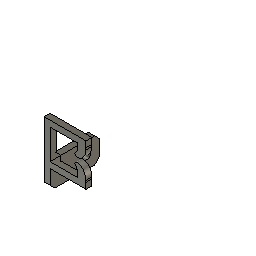
horizontal (Autodesk Fusion 360 design; units mm, degrees)
Autodesk Fusion 360 part; units mm, degrees
sketch "rail-body" plane through (1.3, 0, 0) normal (1, 0, 0) x (0, 1, 0)
  line L0 (50.85, 4.575) -> (60, 4.575)
  line L1 (60, 4.575) -> (60, 14.775)
  line L2 (60, 14.775) -> (0, 14.775)
  line L3 (0, 14.775) -> (0, -14.775)
  line L4 (0, -14.775) -> (60, -14.775)
  line L5 (60, -14.775) -> (60, -4.575)
  line L6 (60, -4.575) -> (50.85, -4.575)
  line L7 (50.85, -4.575) -> (50.85, 4.575)
  line L8 (30.85, 4.575) -> (40, 4.575)
  line L9 (40, 4.575) -> (40, -4.575)
  line L10 (40, -4.575) -> (30.85, -4.575)
  line L11 (30.85, -4.575) -> (30.85, 4.575)
  line L12 (10.85, 4.575) -> (20, 4.575)
  line L13 (20, 4.575) -> (20, -4.575)
  line L14 (20, -4.575) -> (10.85, -4.575)
  line L15 (10.85, -4.575) -> (10.85, 4.575)
  circle A0 centre (15.425, 0) radius 3.5
  line L16 (10.85, 4.575) -> (20, -4.575) construction
  line L17 (20, 4.575) -> (10.85, -4.575) construction
  line L18 (30.85, 4.575) -> (40, -4.575) construction
  line L19 (40, 4.575) -> (30.85, -4.575) construction
  circle A1 centre (35.425, 0) radius 3.5
  line L20 (4.85, 10.575) -> (46, 10.575)
  line L21 (46, 10.575) -> (46, -10.575)
  line L22 (46, -10.575) -> (4.85, -10.575)
  line L23 (4.85, -10.575) -> (4.85, 10.575)
  point P0 (15.425, 0)
  point P1 (35.425, 0)
  dimension "d28" = 7
  dimension "d30" = 7
  dimension "d31" = 6
  dimension "d32" = 6
  dimension "d33" = 6
  dimension "d34" = 6
  constraint coincident L12.start L15.end
  constraint coincident L13.end L14.start
  constraint coincident L12.end L13.start
  constraint coincident L14.end L15.start
  constraint midpoint L16 P0
  constraint coincident P0 A0.centre
  constraint coincident L8.start L11.end
  constraint coincident L9.end L10.start
  constraint coincident L8.end L9.start
  constraint coincident L10.end L11.start
  constraint midpoint L18 P1
  constraint coincident P1 A1.centre
  constraint horizontal L20
  constraint vertical L21
  constraint horizontal L22
  constraint vertical L23
  measures "d28" diameter of A0
  measures "d30" diameter of A1
  measures "d31" distance of L15 L23
  measures "d32" distance of L9 L21
  measures "d33" distance of L14 L22
  measures "d34" distance of L12 L20
extrude "Extrude1" add sketch "rail-body" along normal blind 5 contours L8 L9 L10 L11 | L12 L13 L14 L15 | L20 L21 L22 L23
sketch "cable-body" plane through (0, 4.85, 0) normal (0, -1, 0) x (1, 0, 0)
  line L0 (1.3, 10.575) -> (1.3, -10.575)
  line L1 (1.3, -10.575) -> (6.3, -10.575)
  line L2 (6.3, -10.575) -> (6.3, 10.575)
  line L3 (6.3, 10.575) -> (1.3, 10.575)
  line L4 (6.3, 3.5) -> (6.3, -3.5)
  line L5 (6.3, 5.5) -> (36.3, 5.5)
  line L6 (1.3, 40.5) -> (36.3, 40.5)
  line L7 (6.3, 35.5) -> (36.3, 35.5)
  line L8 (6.3, 10.5) -> (6.3, 35.5)
  line L9 (6.3, 10.5) -> (36.3, 10.5)
  line L10 (1.3, 5.5) -> (1.3, 40.5)
  line L11 (36.3, 5.5) -> (36.3, 10.5)
  line L12 (36.3, 35.5) -> (36.3, 40.5)
  line L13 (6.3, 5.5) -> (1.3, 5.5) construction
  dimension "d51" = 2
  dimension "d53" = 35
  dimension "d55" = 35
  dimension "d56" = 5
  dimension "d57" = 5
  dimension "d58" = 5
  dimension "d59" = 35
  constraint coincident L2 L5.start
  constraint perpendicular L2 L5
  constraint parallel L6 L7
  constraint parallel L5 L9
  constraint vertical L10
  constraint coincident L0 L10.start
  constraint perpendicular L9 L11
  constraint perpendicular L6 L12
  constraint perpendicular L0 L13
  constraint coincident L10.start L13.end
  measures "d51" distance of L4.start L5.start
  measures "d53" distance of L0 L5.end
  measures "d55" distance of L10.start L6.start
  measures "d56" distance of L8 L10
  measures "d57" distance of L6 L7
  measures "d58" distance of L5 L9
  measures "d59" distance of L10 L12
sketch "hook-profile" plane through (0, 0, 0) normal (0, 1, 0) x (1, 0, 0)
  line L0 (6.3, -35.5) -> (36.3, -35.5)
  line L1 (36.3, -35.5) -> (36.3, -40.5)
  line L2 (6.3, -10.5) -> (6.3, -35.5)
  line L3 (6.3, -23) -> (36.2838, -23) construction
  line L4 (29.5303, -34) -> (36.3, -34)
  spline S0 degree 5 poles (36.3, -34) (36.2969, -33.8937) (36.2885, -33.6812) (36.2691, -33.3623) (36.2293, -32.9375) (36.1547, -32.4091) (36.0533, -31.8865) (35.9239, -31.373) (35.7665, -30.8717) (35.5835, -30.3849) (35.3795, -29.9139) (35.1598, -29.4591) (34.9292, -29.0202) (34.6901, -28.597) (34.4418, -28.1889) (34.1783, -27.7958) (33.8908, -27.4178) (33.5695, -27.0553) (33.2063, -26.7097) (32.7967, -26.3826) (32.3428, -26.0767) (31.8525, -25.7957) (31.3377, -25.5438) (30.8125, -25.3262) (30.291, -25.1489) (29.7863, -25.0187) (29.3079, -24.9432) (28.8625, -24.9299) (28.455, -24.9841) (28.0897, -25.108) (27.7716, -25.2988) (27.5068, -25.5475) (27.3024, -25.8403) (27.1648, -26.1605) (27.0993, -26.4904) (27.1085, -26.813) (27.1914, -27.1155) (27.3423, -27.3932) (27.5486, -27.6536) (27.7911, -27.9174) (28.0485, -28.2097) (28.3012, -28.5519) (28.5353, -28.9539) (28.7465, -29.4066) (28.936, -29.8899) (29.1067, -30.3823) (29.2596, -30.8681) (29.3893, -31.3469) (29.4813, -31.841) (29.5355, -32.3554) (29.5566, -32.8899) (29.554, -33.3294) (29.5446, -33.6634) (29.5355, -33.8876) (29.5303, -34) knots 0 0 0 0 0 0 0.02 0.04 0.06 0.08 0.1 0.12 0.14 0.16 0.18 0.2 0.22 0.24 0.26 0.28 0.3 0.32 0.34 0.36 0.38 0.4 0.42 0.44 0.46 0.48 0.5 0.52 0.54 0.56 0.58 0.6 0.62 0.64 0.66 0.68 0.7 0.72 0.74 0.76 0.78 0.8 0.82 0.84 0.86 0.88 0.9 0.92 0.94 0.96 0.98 1 1 1 1 1 1
  line L5 (36.3614, -36.1245) -> (36.2386, -31.8755)
  line L6 (28.7615, -29.0469) -> (29.842, -33.0275)
  line L7 (29.6357, -31.738) -> (29.4248, -36.262)
  line L8 (29.5815, -35.5) -> (36.2971, -35.5)
  line L9 (36.3, -35.5) -> (36.3, -33.7789)
  line L10 (29.5303, -34) -> (29.5303, -35.5)
  point P0 (27.3103, -27.3155)
  point P1 (34.6614, -28.5561)
  point P2 (28.2897, -28.5561)
  point P3 (33.0561, -26.5973)
  point P4 (35.8142, -31.0372)
  point P5 (27.1797, -26.1729)
  point P6 (30.1832, -25.1282)
  point P7 (28.0938, -25.1282)
  point P8 (29.3018, -31.0372)
  dimension "d60" = 1.5
  constraint midpoint L2 L3.start
  constraint perpendicular L2 L3
  constraint coincident L4.start S0.end
  constraint horizontal L4
  constraint midpoint L4.end L5
  constraint midpoint P8 L6
  constraint midpoint L4.start L7
  constraint horizontal L8
  constraint collinear L0 L8
  constraint coincident L0.end L1.start
  constraint perpendicular L8 L9
  constraint coincident L4.end L9
  constraint coincident L0 L10.end
  constraint vertical L10
  measures "d60" distance of L4 L8
sketch "Sketch5" plane through (3.8, 4.85, 0) normal (0, -1, 0) x (1, 0, 0)
  line L0 (2.5, 35.5) -> (32.5, 35.5)
  line L1 (2.5, 10.5) -> (2.5, 35.5)
  line L2 (-2.5, 40.5) -> (32.5, 40.5)
  line L3 (32.5, 35.5) -> (32.5, 40.5)
  line L4 (-2.5, 5.5) -> (-2.5, 40.5)
  line L5 (2.5, 5.5) -> (-2.5, 5.5)
  line L6 (2.5, 5.5) -> (32.5, 5.5)
  line L7 (32.5, 5.5) -> (32.5, 10.5)
  line L8 (2.5, 10.5) -> (32.5, 10.5)
  spline S0 degree 5 poles (36.3, -34) (36.2969, -33.8937) (36.2885, -33.6812) (36.2691, -33.3623) (36.2293, -32.9375) (36.1547, -32.4091) (36.0533, -31.8865) (35.9239, -31.373) (35.7665, -30.8717) (35.5835, -30.3849) (35.3795, -29.9139) (35.1598, -29.4591) (34.9292, -29.0202) (34.6901, -28.597) (34.4418, -28.1889) (34.1783, -27.7958) (33.8908, -27.4178) (33.5695, -27.0553) (33.2063, -26.7097) (32.7967, -26.3826) (32.3428, -26.0767) (31.8525, -25.7957) (31.3377, -25.5438) (30.8125, -25.3262) (30.291, -25.1489) (29.7863, -25.0187) (29.3079, -24.9432) (28.8625, -24.9299) (28.455, -24.9841) (28.0897, -25.108) (27.7716, -25.2988) (27.5068, -25.5475) (27.3024, -25.8403) (27.1648, -26.1605) (27.0993, -26.4904) (27.1085, -26.813) (27.1914, -27.1155) (27.3423, -27.3932) (27.5486, -27.6536) (27.7911, -27.9174) (28.0485, -28.2097) (28.3012, -28.5519) (28.5353, -28.9539) (28.7465, -29.4066) (28.936, -29.8899) (29.1067, -30.3823) (29.2596, -30.8681) (29.3893, -31.3469) (29.4813, -31.841) (29.5355, -32.3554) (29.5566, -32.8899) (29.554, -33.3294) (29.5446, -33.6634) (29.5355, -33.8876) (29.5303, -34) knots 0 0 0 0 0 0 0.02 0.04 0.06 0.08 0.1 0.12 0.14 0.16 0.18 0.2 0.22 0.24 0.26 0.28 0.3 0.32 0.34 0.36 0.38 0.4 0.42 0.44 0.46 0.48 0.5 0.52 0.54 0.56 0.58 0.6 0.62 0.64 0.66 0.68 0.7 0.72 0.74 0.76 0.78 0.8 0.82 0.84 0.86 0.88 0.9 0.92 0.94 0.96 0.98 1 1 1 1 1 1
  line L9 (36.3614, -36.1245) -> (36.2386, -31.8755)
  line L10 (28.7615, -29.0469) -> (29.842, -33.0275)
  line L11 (29.6357, -31.738) -> (29.4248, -36.262)
  spline S1 degree 5 poles (32.5, 34) (32.4969, 33.8937) (32.4885, 33.6812) (32.4691, 33.3623) (32.4293, 32.9375) (32.3547, 32.4091) (32.2533, 31.8865) (32.1239, 31.373) (31.9665, 30.8717) (31.7835, 30.3849) (31.5795, 29.9139) (31.3598, 29.4591) (31.1292, 29.0202) (30.8901, 28.597) (30.6418, 28.1889) (30.3783, 27.7958) (30.0908, 27.4178) (29.7695, 27.0553) (29.4063, 26.7097) (28.9967, 26.3826) (28.5428, 26.0767) (28.0525, 25.7957) (27.5377, 25.5438) (27.0125, 25.3262) (26.491, 25.1489) (25.9863, 25.0187) (25.5079, 24.9432) (25.0625, 24.9299) (24.655, 24.9841) (24.2897, 25.108) (23.9716, 25.2988) (23.7068, 25.5475) (23.5024, 25.8403) (23.3648, 26.1605) (23.2993, 26.4904) (23.3085, 26.813) (23.3914, 27.1155) (23.5423, 27.3932) (23.7486, 27.6536) (23.9911, 27.9174) (24.2485, 28.2097) (24.5012, 28.5519) (24.7353, 28.9539) (24.9465, 29.4066) (25.136, 29.8899) (25.3067, 30.3823) (25.4596, 30.8681) (25.5893, 31.3469) (25.6813, 31.841) (25.7355, 32.3554) (25.7566, 32.8899) (25.754, 33.3294) (25.7446, 33.6634) (25.7355, 33.8876) (25.7303, 34) knots 0 0 0 0 0 0 0.02 0.04 0.06 0.08 0.1 0.12 0.14 0.16 0.18 0.2 0.22 0.24 0.26 0.28 0.3 0.32 0.34 0.36 0.38 0.4 0.42 0.44 0.46 0.48 0.5 0.52 0.54 0.56 0.58 0.6 0.62 0.64 0.66 0.68 0.7 0.72 0.74 0.76 0.78 0.8 0.82 0.84 0.86 0.88 0.9 0.92 0.94 0.96 0.98 1 1 1 1 1 1
  line L12 (25.7303, 34) -> (25.7303, 35.5)
  line L13 (32.5, 35.5) -> (32.5, 33.7789)
  line L14 (2.5, 23) -> (32.4838, 23)
  spline S2 degree 5 poles (32.5, 12) (32.4969, 12.1063) (32.4885, 12.3188) (32.4691, 12.6377) (32.4293, 13.0625) (32.3547, 13.5909) (32.2533, 14.1135) (32.1239, 14.627) (31.9665, 15.1283) (31.7835, 15.6151) (31.5795, 16.0861) (31.3598, 16.5409) (31.1292, 16.9798) (30.8901, 17.403) (30.6418, 17.8111) (30.3783, 18.2042) (30.0908, 18.5822) (29.7695, 18.9447) (29.4063, 19.2903) (28.9967, 19.6174) (28.5428, 19.9233) (28.0525, 20.2043) (27.5377, 20.4562) (27.0125, 20.6738) (26.491, 20.8511) (25.9863, 20.9813) (25.5079, 21.0568) (25.0625, 21.0701) (24.655, 21.0159) (24.2897, 20.892) (23.9716, 20.7012) (23.7068, 20.4525) (23.5024, 20.1597) (23.3648, 19.8395) (23.2993, 19.5096) (23.3085, 19.187) (23.3914, 18.8845) (23.5423, 18.6068) (23.7486, 18.3464) (23.9911, 18.0826) (24.2485, 17.7903) (24.5012, 17.4481) (24.7353, 17.0461) (24.9465, 16.5934) (25.136, 16.1101) (25.3067, 15.6177) (25.4596, 15.1319) (25.5893, 14.6531) (25.6813, 14.159) (25.7355, 13.6446) (25.7566, 13.1101) (25.754, 12.6706) (25.7446, 12.3366) (25.7355, 12.1124) (25.7303, 12) knots 0 0 0 0 0 0 0.02 0.04 0.06 0.08 0.1 0.12 0.14 0.16 0.18 0.2 0.22 0.24 0.26 0.28 0.3 0.32 0.34 0.36 0.38 0.4 0.42 0.44 0.46 0.48 0.5 0.52 0.54 0.56 0.58 0.6 0.62 0.64 0.66 0.68 0.7 0.72 0.74 0.76 0.78 0.8 0.82 0.84 0.86 0.88 0.9 0.92 0.94 0.96 0.98 1 1 1 1 1 1
  line L15 (32.5, 10.5) -> (32.5, 12.2211)
  line L16 (25.7303, 12) -> (25.7303, 10.5)
  point P0 (29.3018, -31.0372)
  point P1 (27.1797, -26.1729)
  point P2 (28.0938, -25.1282)
  point P3 (30.1832, -25.1282)
  point P4 (35.8142, -31.0372)
  point P5 (33.0561, -26.5973)
  point P6 (34.6614, -28.5561)
  point P7 (27.3103, -27.3155)
  point P8 (28.2897, -28.5561)
  constraint midpoint S0.start L9
  constraint midpoint P0 L10
  constraint midpoint S0.end L11
  constraint symmetric S1.start L14 S2.start
  constraint symmetric S1.end L14 S2.end
  constraint symmetric S1 L14 S2
  constraint symmetric L12.end L14 L16.end
  constraint symmetric L0.end L14 L7.end
  constraint symmetric L13.end L14 L15.end
extrude "Extrude2" add sketch "cable-body" sketch "Sketch5" against normal blind 5 contours L3 L6 L7 L8 L10 L12 of sketch 2 contours L0 L1 L2 L3 L4 L5 L6 L7 L8 | L0 S1 L12 L13 | L8 S2 L15 L16
chamfer "Chamfer1" distance 4 angle 45 2 edges at (3.8, 9.85, 10.575) (6.3, 9.85, 8)
chamfer "Chamfer2" distance 4 angle 45 3 edges at (3.8, 4.85, -10.575) (3.8, 46, -10.575) (3.8, 46, 10.575)
equation "d30 = d28"
equation "d32 = d31"
equation "d34 = d33"
equation "d53 = d55"
equation "d57 = d56"
equation "d58 = d56"
equation "d59 = d55"
